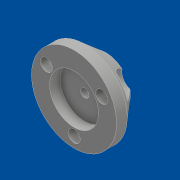
# Autodesk Inventor part: 902-4250 magnet hold
Saved by Autodesk Inventor 2018 (Build 220112000, 112)
## iProperties
Created: 2019-12-10
Part Number: 902-4250 magnet hold
Material: Generic
Document SubType Name: Modeling
Designer: Bunny320
Density: 1 g/cm^3
Appearance: Light Gray
Author: Bunny320
## iProperties of the stored document 922-2820 magnet hold_3DPrint.ipt
Created: 2020-06-14
Part Number: 922-2820 magnet hold_3DPrint
Material: Generic
Document SubType Name: Modeling
Designer: Bunny320
Density: 1 g/cm^3
Appearance: Default
Author: Bunny320
Autodesk Inventor part; units mm, degrees
ref_plane "YZ Plane" through (0, 0, 0) normal (1, 0, 0) x (0, 1, 0)
ref_plane "XZ Plane" through (0, 0, 0) normal (0, 1, 0) x (-1, 0, 0)
ref_plane "XY Plane" through (0, 0, 0) normal (0, 0, 1) x (1, 0, 0)
sketch "Sketch2" plane through (0, 0, 0) normal (0, 0, 1) x (1, 0, 0)
  line L0 (1, 2.5) -> (1, 5.5)
  line L1 (1, 5.5) -> (3, 5.5)
  line L2 (3, 5.5) -> (3, 7.5)
  line L3 (3, 7.5) -> (5.75, 7.5)
  line L4 (5.75, 7.5) -> (10, 2.5)
  line L5 (10, 2.5) -> (10, 0)
  line L6 (1, 2.5) -> (5.75, 2.5)
  line L7 (5.75, 2.5) -> (5.75, 0)
  line L8 (5.75, 0) -> (10, 0)
  line L9 (0, 0) -> (0, 19.425)
  dimension "d0" = 6
  dimension "d1" = 2
  dimension "d2" = 11.5
  dimension "d3" = 20
  dimension "d4" = 2.5
  dimension "d5" = 3
  dimension "d6" = 2
  constraints: 20 end point, 5 perpendicular, 3 point on line, 2 vertical, 1 horizontal, 1 parallel
  measures "d0" diameter of L2 L9
  measures "d1" diameter of L0 L9
  measures "d2" diameter of L7 L9
  measures "d3" diameter of L5 L9
  measures "d4" distance of L6.end L7.end
  measures "d5" distance of L0.start L0.end
  measures "d6" distance of L1.end L2.end
revolve "Revolution1" add sketch "Sketch2" angle 360 about axis through (0, 0, 0) along (0, 1, 0)
sketch "Sketch3" plane through (0, 7.5, 0) normal (0, 1, 0) x (1, 0, 0)
  point P0 (0, 0)
  point P1 (0, 7.5)
  dimension "d8" = 7.5
  constraints: 1 vertical alignment
  measures "d8" distance of point (0, 0) point (0, 7.5)
hole "Hole1" at (0, 7.5, -7.5) direction (0, -1, 0) diameter 2.9 end through all counterbore diameter 5.5 counterbore depth 3.5 clearance for "Socket Head Cap Screw DIN EN ISO 4762" size "M2.5" standard "DIN"
pattern_circular "Circular Pattern1" count 3 over 360 about axis through (0, -10, 0) along (0, 1, 0) of "Hole1"
body "Solid1"
